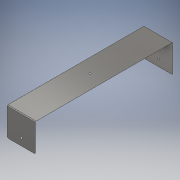
# Autodesk Inventor part: Part9
Saved by Autodesk Inventor 2019 (Build 230136000, 136)
## iProperties
Created: 2019-08-22
Part Number: Part9
Material: Iron, Malleable
Document SubType Name: Modeling
Designer: bowen.wu2
Density: 7.15 g/cm^3
Appearance: Semi-Polished
Author: bowen.wu2
Autodesk Inventor part; units mm, degrees
ref_plane "YZ Plane" through (0, 0, 0) normal (1, 0, 0) x (0, 1, 0)
ref_plane "XY Plane" through (0, 0, 0) normal (0, 0, 1) x (1, 0, 0)
sketch "Sketch1" plane through (0, 0, 0) normal (1, 0, 0) x (0, 1, 0)
  line L0 (20, 97) -> (-20, 97) construction
  line L1 (-20, 97) -> (-20, -97) construction
  line L2 (-20, -97) -> (20, -97) construction
  line L3 (20, -97) -> (20, 97) construction
  line L4 (20, 97) -> (-20, -97) construction
  line L5 (-20, 97) -> (20, -97) construction
  line L6 (-20, 97) -> (19, 97)
  line L7 (-20, -97) -> (19, -97)
  arc A0 (20, 95.9982) -> (19, 97) centre (19, 96) ccw
  arc A1 (19, -97) -> (20, -95.9993) centre (19, -96) ccw
  line L8 (20, 95.9982) -> (20, -95.9993)
  point P0 (0, 0)
  dimension "d0" = 40
  dimension "d1" = 194
  dimension "d2" = 39
  dimension "d3" = 39
  constraints: 18 end point, 4 point on circle, 4 point on line, 2 centre point, 2 midpoint, 2 parallel, 2 tangent, 1 horizontal, 1 perpendicular
  measures "d0" distance of L2.end L1.end
  measures "d1" distance of L1.end L0.end
  measures "d2" distance of L0.end L6.end
  measures "d3" distance of L1.end L7.end
ref_plane "Work Plane1" through (0, -20, 97) normal (0, 1, 0) x (-1, 0, 0)
sketch "Sketch2" plane through (0, -20, 97) normal (0, 1, 0) x (-1, 0, 0)
  line L0 (0, 0) -> (40, 0)
  line L1 (40, 0) -> (40, -0.1)
  line L2 (40, -0.1) -> (0, -0.1)
  line L3 (0, -0.1) -> (0, 0)
  point P0 (0, -97)
  dimension "d4" = 40
  dimension "d5" = 0.1
  constraints: 8 end point, 2 parallel, 1 horizontal, 1 perpendicular
  measures "d4" distance of L1.end L2.end
  measures "d5" distance of L0.end L1.end
sweep "Sweep1" add profiles "Sketch2" path "Sketch1" path curves L6 A0 L8 A1 L7
sketch "Sketch3" plane through (-40, 20, 95.9982) normal (0, 1, 0) x (1, 0, 0)
  line L0 (0, -0.0002) -> (0, 191.9975) construction
  line L1 (40, 0) -> (40, -1.0018) construction
  line L2 (0, 191.9975) -> (40, 0) construction
  line L3 (40, -0.0002) -> (40, 191.9975) construction
  line L4 (40, 191.9975) -> (0, -0.0002) construction
  point P0 (40, 95.9982)
  point P1 (20, 95.9987)
  constraints: 4 end point, 1 midpoint
hole "Hole1" at (-20, 20, -0.0004) direction (0, -1, 0) diameter 3 end through all
fillet "Fillet1" radius 2 4 edges at (0, -20, 96.95) (-40, -20, 96.95) (0, -19.9999, -96.95) (-40, -19.9999, -96.95)
sketch "Sketch4" plane through (-40, 19, 97) normal (0, 0, 1) x (1, 0, 0)
  line L0 (0, -37) -> (0, 0) projected
  line L1 (38, -39) -> (2, -39) projected
  point P0 (40, -19)
  point P1 (20, -29)
  dimension "d16" = 20
  dimension "d17" = 10
  measures "d16" distance from line of point (20, -29) L0
  measures "d17" distance from line of L1 point (20, -29)
hole "Hole2" at (-20, -10, 97) direction (0, 0, -1) diameter 3 end through all
equation "\"d3\" = d2"
body "Solid1"
